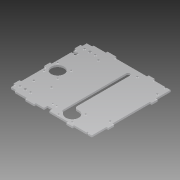
# Autodesk Inventor part: plastic_part_04
Saved by Autodesk Inventor 2013 (Build 170138000, 138)
## iProperties
Shininess: 20.0
Created: 2013-02-12
Part Number: plastic_part_04
Document SubType Name: Modeling
Designer: Noa Izumi
Material: Default
Density: 1 g/cm^3
Density: 0.0
Volumn: 0.0
Area: 0.0
PropertySet Name: Model Information
Control State: 0
Master: False
Checked Out: False
Author: Noa Izumi
Autodesk Inventor part; units mm, degrees
ref_plane "YZ Plane" through (0, 0, 0) normal (1, 0, 0) x (0, 1, 0)
ref_plane "XZ Plane" through (0, 0, 0) normal (0, 1, 0) x (-1, 0, 0)
ref_plane "XY Plane" through (0, 0, 0) normal (0, 0, 1) x (1, 0, 0)
sketch "Sketch1" plane through (0, 0, 0) normal (0, 0, 1) x (1, 0, 0)
  line L0 (0, 0) -> (140, 0)
  line L1 (140, 0) -> (140, 134)
  line L2 (140, 134) -> (0, 134)
  line L3 (0, 134) -> (0, 0)
  line L4 (30, 137) -> (45, 137)
  line L5 (45, 137) -> (45, -3)
  line L6 (45, -3) -> (30, -3)
  line L7 (30, -3) -> (30, 137)
  line L8 (100, 137) -> (110, 137)
  line L9 (110, 137) -> (110, -3)
  line L10 (110, -3) -> (100, -3)
  line L11 (100, -3) -> (100, 137)
  line L12 (-3, 124) -> (0, 124)
  line L13 (0, 124) -> (0, 114)
  line L14 (0, 114) -> (-3, 114)
  line L15 (-3, 114) -> (-3, 124)
  line L16 (-3, 20) -> (0, 20)
  line L17 (0, 20) -> (0, 10)
  line L18 (0, 10) -> (-3, 10)
  line L19 (-3, 10) -> (-3, 20)
  line L20 (-3, 72) -> (0, 72)
  line L21 (0, 72) -> (0, 62)
  line L22 (0, 62) -> (-3, 62)
  line L23 (-3, 62) -> (-3, 72)
  line L24 (140, 109) -> (143, 109)
  line L25 (143, 109) -> (143, 99)
  line L26 (143, 99) -> (140, 99)
  line L27 (140, 99) -> (140, 109)
  line L28 (140, 35) -> (143, 35)
  line L29 (143, 35) -> (143, 25)
  line L30 (143, 25) -> (140, 25)
  line L31 (140, 25) -> (140, 35)
  dimension "d0" = 140
  dimension "d1" = 134
  dimension "d2" = 140
  dimension "d3" = 3
  dimension "d4" = 15
  dimension "d5" = 10
  dimension "d6" = 140
  dimension "d7" = 3
  dimension "d8" = 30
  dimension "d9" = 30
  dimension "d10" = 10
  dimension "d12" = 3
  dimension "d13" = 10
  dimension "d14" = 3
  dimension "d15" = 3
  dimension "d16" = 10
  dimension "d17" = 10
  dimension "d103" = 10
  dimension "d104" = 42
  dimension "d208" = 3
  dimension "d213" = 3
  dimension "d214" = 10
  dimension "d215" = 25
  dimension "d216" = 3
  dimension "d217" = 10
  dimension "d218" = 25
  constraints: 64 end point, 16 parallel, 8 horizontal, 8 perpendicular, 2 point on line
  measures "d0" distance of L0.start L0.end
  measures "d1" distance of L2.end L0.start
  measures "d2" distance of L6.end L4.start
  measures "d3" distance between parallel lines of L6 L0
  measures "d4" distance of L5.end L6.end
  measures "d5" distance of L9.end L10.end
  measures "d6" distance of L8.end L9.end
  measures "d7" distance between parallel lines of L10 L0
  measures "d8" distance between parallel lines of L7 L3
  measures "d9" distance between parallel lines of L1 L9
  measures "d10" distance of L14.end L12.start
  measures "d12" distance between parallel lines of L3 L15
  measures "d13" distance of L18.end L16.start
  measures "d14" distance between parallel lines of L3 L19
  measures "d15" distance of L17.end L18.end
  measures "d16" distance between parallel lines of L2 L12
  measures "d17" distance between parallel lines of L0 L18
  measures "d103" distance of L22.end L20.start
  measures "d104" distance between parallel lines of L20 L14
  measures "d208" distance of L21.end L22.end
  measures "d213" distance of L24.start L24.end
  measures "d214" distance of L24.end L25.end
  measures "d215" distance between parallel lines of L24 L2
  measures "d216" distance between parallel lines of L29 L31
  measures "d217" distance of L28.end L29.end
  measures "d218" distance between parallel lines of L30 L0
extrude "Extrusion1" add sketch "Sketch1" along normal blind 3
sketch "Sketch2" plane through (0, 0, 3) normal (0, 0, 1) x (1, 0, 0)
  line L0 (0, 0) -> (0, 10) projected
  line L1 (100, 0) -> (45, 0) projected
  point P0 (80.25, 3.5)
  point P1 (103.25, 26.5)
  point P2 (103.25, 3.5)
  dimension "d102" = 23
  dimension "d119" = 80.25
  dimension "d122" = 3.5
  dimension "d123" = 23
  measures "d102" distance of point (103.25, 3.5) point (80.25, 3.5)
  measures "d119" distance from line of point (80.25, 3.5) L0
  measures "d122" distance from line of L1 point (80.25, 3.5)
  measures "d123" distance of point (103.25, 26.5) point (103.25, 3.5)
hole "Hole1" at (80.25, 3.5, 3) at (103.25, 26.5, 3) at (103.25, 3.5, 3) direction (0, 0, -1) diameter 2.5 end through all
sketch "Sketch3" plane through (0, 0, 3) normal (0, 0, 1) x (1, 0, 0)
  line L0 (0, 20) -> (0, 114) projected
  line L1 (30, 0) -> (0, 0) projected
  line L2 (0, 0) -> (0, 10) projected
  point P0 (3.5, 78.5)
  point P1 (3.5, 55.5)
  point P2 (26.5, 78.5)
  point P3 (26.5, 55.5)
  dimension "d35" = 23
  dimension "d37" = 3.5
  dimension "d48" = 3.5
  dimension "d93" = 55.5
  dimension "d101" = 23
  dimension "d105" = 23
  measures "d35" distance of point (3.5, 55.5) point (3.5, 78.5)
  measures "d37" distance from line of L0 point (3.5, 78.5)
  measures "d48" distance from line of point (3.5, 55.5) L2
  measures "d93" distance from line of L1 point (3.5, 55.5)
  measures "d101" distance of point (3.5, 78.5) point (26.5, 78.5)
  measures "d105" distance of point (26.5, 55.5) point (3.5, 55.5)
hole "Hole2" at (3.5, 78.5, 3) at (3.5, 55.5, 3) at (26.5, 78.5, 3) at (26.5, 55.5, 3) direction (0, 0, -1) diameter 2.5 end through all
sketch "Sketch5" plane through (0, 0, 3) normal (0, 0, 1) x (1, 0, 0)
  line L0 (0, 124) -> (0, 134) projected
  line L1 (0, 0) -> (0, 10) projected
  line L2 (0, 134) -> (30, 134) projected
  line L3 (30, 0) -> (0, 0) projected
  point P0 (15, 122)
  point P1 (15, 12)
  dimension "d56" = 15
  dimension "d57" = 15
  dimension "d89" = 12
  dimension "d90" = 12
  measures "d56" distance from line of L0 point (15, 122)
  measures "d57" distance from line of L1 point (15, 12)
  measures "d89" distance from line of L3 point (15, 12)
  measures "d90" distance from line of point (15, 122) L2
hole "Hole3" at (15, 122, 3) at (15, 12, 3) direction (0, 0, -1) diameter 4 end through all
sketch "Sketch6" plane through (0, 0, 3) normal (0, 0, 1) x (1, 0, 0)
  circle A0 centre (15, 122) radius 2 projected
  circle A1 centre (15, 12) radius 2 projected
  point P0 (6, 122)
  point P1 (24, 122)
  point P2 (6, 12)
  point P3 (24, 12)
  dimension "d65" = 9
  dimension "d66" = 9
  dimension "d67" = 9
  dimension "d68" = 9
  dimension "d91" = 0
  dimension "d92" = 0
  measures "d65" distance of A0.centre point (6, 122)
  measures "d66" distance of point (24, 122) A0.centre
  measures "d67" distance of A1.centre point (6, 12)
  measures "d68" distance of A1.centre point (24, 12)
  measures "d91" vertical distance of A1.centre point (6, 12)
  measures "d92" vertical distance of A0.centre point (6, 122)
hole "Hole4" at (6, 122, 3) at (24, 122, 3) at (6, 12, 3) at (24, 12, 3) direction (0, 0, -1) diameter 3 end through all
sketch "Sketch8" plane through (0, 0, 3) normal (0, 0, 1) x (1, 0, 0)
  line L0 (45, 134) -> (100, 134) projected
  line L1 (140, 134) -> (140, 109) projected
  point P0 (92, 125.5)
  dimension "d136" = 8.5
  dimension "d226" = 48
  measures "d136" distance from line of point (92, 125.5) L0
  measures "d226" distance from line of L1 point (92, 125.5)
hole "Hole5" at (92, 125.5, 3) direction (0, 0, -1) diameter 3 end through all
sketch "Sketch13" plane through (0, 0, 3) normal (0, 0, 1) x (1, 0, 0)
  circle A0 centre (3.5, 78.5) radius 1.25 projected
  circle A1 centre (80.25, 3.5) radius 1.25 projected
  point P0 (15, 67)
  point P1 (91.75, 15)
  dimension "d108" = 11.5
  dimension "d109" = 11.5
  dimension "d124" = 11.5
  dimension "d125" = 11.5
  measures "d108" horizontal distance of point (15, 67) A0.centre
  measures "d109" horizontal distance of A0.centre point (15, 67)
  measures "d124" horizontal distance of point (91.75, 15) A1.centre
  measures "d125" horizontal distance of point (91.75, 15) A1.centre
hole "Hole6" at (15, 67, 3) at (91.75, 15, 3) direction (0, 0, -1) diameter 22 end through all
sketch "Sketch15" plane through (0, 0, 3) normal (0, 0, 1) x (1, 0, 0)
  line L0 (100, 0) -> (45, 0) projected
  line L1 (45, 134) -> (100, 134) projected
  line L2 (81, 124) -> (81, 124)
  line L3 (84.25, 120.75) -> (84.25, 10)
  line L4 (84.25, 10) -> (81, 10)
  line L5 (77.75, 13.25) -> (77.75, 120.75)
  arc A0 (81, 124) -> (77.75, 120.75) centre (81, 120.75) ccw
  arc A1 (84.25, 120.75) -> (81, 124) centre (81, 120.75) ccw
  arc A2 (77.75, 13.25) -> (81, 10) centre (81, 13.25) ccw
  circle A3 centre (91.75, 15) radius 11 projected
  point P0 (77.75, 124)
  point P1 (84.25, 124)
  point P2 (77.75, 10)
  dimension "d129" = 10
  dimension "d130" = 6.5
  dimension "d131" = 3.25
  dimension "d137" = 10
  dimension "d138" = 3.25
  dimension "d224" = 14
  constraints: 8 end point, 6 point on circle, 6 point on line, 6 tangent, 3 centre point, 2 parallel, 1 concentric, 1 horizontal, 1 perpendicular
  measures "d129" distance between parallel lines of L0 L4
  measures "d130" distance of point (77.75, 124) point (84.25, 124)
  measures "d131" radius of A0
  measures "d137" distance from line of L1 L2.end
  measures "d138" radius of A2
  measures "d224" distance from line of A3.centre L5
extrude "Extrusion2" cut sketch "Sketch15" against normal through all contours L3 A3 L4 A2 L5 A0 A1 | L3 L4 A3 picked at (83.7345, 18.1015)
sketch "Sketch19" plane through (0, 0, 3) normal (0, 0, 1) x (1, 0, 0)
  line L0 (140, 0) -> (110, 0) projected
  line L1 (110, 134) -> (140, 134) projected
  line L2 (133.3, 134) -> (131, 134)
  line L3 (131, 134) -> (131, 132.25)
  line L4 (131, 132.25) -> (133.3, 132.25)
  line L5 (133.3, 132.25) -> (133.3, 134)
  line L6 (133.3, 0) -> (131, 0)
  line L7 (131, 0) -> (131, 1.75)
  line L8 (131, 1.75) -> (133.3, 1.75)
  line L9 (133.3, 1.75) -> (133.3, 0)
  line L10 (140, 134) -> (140, 0) projected
  line L11 (0, 134) -> (9.175, 134)
  line L12 (9.175, 134) -> (9.175, 132.75)
  line L13 (7.925, 131.5) -> (0, 131.5)
  line L14 (0, 131.5) -> (0, 134)
  line L15 (0, 0) -> (9.175, 0)
  line L16 (9.175, 0) -> (9.175, 1.25)
  line L17 (7.925, 2.5) -> (0, 2.5)
  line L18 (0, 2.5) -> (0, 0)
  arc A0 (7.925, 131.5) -> (9.175, 132.75) centre (7.925, 132.75) ccw
  arc A1 (9.175, 1.25) -> (7.925, 2.5) centre (7.925, 1.25) ccw
  point P0 (9.175, 131.5)
  point P1 (9.175, 2.5)
  dimension "d166" = 2.3
  dimension "d168" = 1.75
  dimension "d173" = 1.75
  dimension "d210" = 9
  dimension "d211" = 2.3
  dimension "d212" = 9
  dimension "d219" = 9.175
  dimension "d220" = 2.5
  dimension "d221" = 9.175
  dimension "d222" = 2.5
  dimension "d223" = 1.25
  constraints: 32 end point, 8 parallel, 6 point on line, 4 horizontal, 4 perpendicular, 4 point on circle, 4 tangent, 2 centre point, 1 equal radius
  measures "d166" distance of L3.end L4.end
  measures "d168" distance of L2.end L3.end
  measures "d173" distance of L6.end L7.end
  measures "d210" distance between parallel lines of L10 L7
  measures "d211" distance of L7.end L8.end
  measures "d212" distance between parallel lines of L10 L3
  measures "d219" distance of point (9.175, 131.5) L13.end
  measures "d220" distance of L11.end point (9.175, 131.5)
  measures "d221" distance of point (9.175, 2.5) L17.end
  measures "d222" distance of L15.end point (9.175, 2.5)
  measures "d223" radius of A0
extrude "Extrusion3" cut sketch "Sketch19" against normal through all
fillet "圓角4" radius 5 2 edges at (84.25, 23.0467, 1.5) (81.952, 10, 1.5)
sketch "草圖24" plane through (0, 0, 3) normal (0, 0, 1) x (1, 0, 0)
  line L0 (140, 0) -> (133.3, 0) projected
  line L1 (140, 99) -> (140, 35) projected
  point P0 (0, 0)
  point P1 (134.5, 37)
  point P2 (34.5, 37)
  point P3 (134.5, 117)
  point P4 (34.5, 117)
  dimension "d227" = 37
  dimension "d228" = 5.5
  dimension "d229" = 100
  dimension "d230" = 80
  measures "d227" distance from line of L0 point (134.5, 37)
  measures "d228" distance from line of L1 point (134.5, 37)
  measures "d229" distance of point (134.5, 37) point (34.5, 37)
  measures "d230" distance of point (134.5, 37) point (134.5, 117)
hole "孔10" at (134.5, 37, 3) at (34.5, 37, 3) at (134.5, 117, 3) at (34.5, 117, 3) direction (0, 0, -1) diameter 3 end through all
sketch "草圖25" plane through (0, 0, 3) normal (0, 0, 1) x (1, 0, 0)
  line L0 (0, 20) -> (0, 62) projected
  line L1 (30, 0) -> (9.175, 0) projected
  point P0 (0, 0)
  point P1 (9.5, 32)
  dimension "d238" = 9.5
  dimension "d239" = 32
  measures "d238" distance from line of point (9.5, 32) L0
  measures "d239" distance from line of L1 point (9.5, 32)
hole "孔11" at (9.5, 32, 3) direction (0, 0, -1) diameter 3 end through all
sketch "草圖26" plane through (0, 0, 3) normal (0, 0, 1) x (1, 0, 0)
  line L0 (0, 72) -> (0, 114) projected
  line L1 (9.175, 134) -> (30, 134) projected
  line L2 (0, 108.5) -> (4.5635, 108.5)
  line L3 (8, 108.5) -> (8, 105.5)
  line L4 (4.5635, 105.5) -> (0, 105.5)
  line L5 (0, 105.5) -> (0, 108.5)
  line L6 (6.5, 110) -> (6.5, 110)
  line L7 (6.5, 104) -> (6.5, 104)
  line L8 (8, 105.5) -> (8, 108.5)
  arc A0 (8, 108.5) -> (6.5, 110) centre (6.5, 108.5) ccw
  arc A1 (6.5, 104) -> (8, 105.5) centre (6.5, 105.5) ccw
  arc A2 (5.0476, 105.125) -> (6.5, 104) centre (6.5, 105.5) ccw
  arc A3 (6.5, 110) -> (5.0476, 108.875) centre (6.5, 108.5) ccw
  arc A4 (4.5635, 108.5) -> (5.0476, 108.875) centre (4.5635, 109) ccw
  arc A5 (5.0476, 105.125) -> (4.5635, 105.5) centre (4.5635, 105) ccw
  point P0 (0, 0)
  point P1 (8, 110)
  point P2 (5, 110)
  point P3 (8, 104)
  point P4 (5, 108.5)
  point P5 (5, 105.5)
  dimension "d249" = 3
  dimension "d250" = 25.5
  dimension "d251" = 3
  dimension "d252" = 6
  dimension "d253" = 8
  dimension "d255" = 1.5
  dimension "d256" = 0.5
  constraints: 14 end point, 14 point on circle, 10 tangent, 8 point on line, 6 centre point, 4 equal radius, 3 parallel, 2 horizontal, 1 perpendicular
  measures "d249" distance of L4.end L2.start
  measures "d250" distance between parallel lines of L2 L1
  measures "d251" distance of point (8, 110) point (5, 110)
  measures "d252" distance of point (8, 104) point (8, 110)
  measures "d253" distance between parallel lines of L8 L0
  measures "d255" radius of A0
  measures "d256" radius of A4
extrude "擠出7" cut sketch "草圖26" against normal through all
sketch "草圖27" plane through (0, 0, 3) normal (0, 0, 1) x (1, 0, 0)
  line L0 (100, 0) -> (45, 0) projected
  line L1 (140, 25) -> (140, 0) projected
  point P0 (0, 0)
  point P1 (66.25, 14)
  point P2 (59.75, 14)
  dimension "d259" = 73.75
  dimension "d260" = 14
  dimension "d261" = 6.5
  measures "d259" distance from line of L1 point (66.25, 14)
  measures "d260" distance from line of L0 point (66.25, 14)
  measures "d261" distance of point (66.25, 14) point (59.75, 14)
hole "孔12" at (66.25, 14, 3) at (59.75, 14, 3) direction (0, 0, -1) diameter 2 end through all
sketch "草圖28" plane through (0, 0, 3) normal (0, 0, 1) x (1, 0, 0)
  circle A0 centre (66.25, 14) radius 1 projected
  line L0 (100, 0) -> (45, 0) projected
  line L1 (59.75, 6) -> (66.75, 6)
  line L2 (67.75, 5) -> (67.75, 0)
  line L3 (67.75, 0) -> (58.75, 0)
  line L4 (58.75, 0) -> (58.75, 5)
  arc A1 (59.75, 6) -> (58.75, 5) centre (59.75, 5) ccw
  arc A2 (67.75, 5) -> (66.75, 6) centre (66.75, 5) ccw
  point P0 (0, 0)
  point P1 (58.75, 6)
  point P2 (67.75, 6)
  dimension "d269" = 6
  dimension "d271" = 9
  dimension "d272" = 1.5
  dimension "d273" = 1
  constraints: 8 end point, 5 point on line, 4 point on circle, 4 tangent, 2 centre point, 2 parallel, 1 equal radius, 1 horizontal, 1 perpendicular
  measures "d269" distance of point (67.75, 6) L2.end
  measures "d271" distance of point (58.75, 6) point (67.75, 6)
  measures "d272" distance from line of L2 A0.centre
  measures "d273" radius of A1
extrude "擠出8" cut sketch "草圖28" against normal through all contours L0 L4 A1 L1 A2 L2
